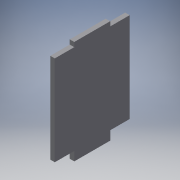
# Autodesk Inventor part: Base and top seperator
Saved by Autodesk Inventor 2018 (Build 220112000, 112)
## iProperties
Created: 2018-05-02
Part Number: Base and top seperator
Material: Generic
Document SubType Name: Modeling
Designer: Ajith Thomas
Density: 1 g/cm^3
Appearance: Default
Author: Ajith Thomas
Autodesk Inventor part; units mm, degrees
ref_plane "YZ Plane" through (0, 0, 0) normal (1, 0, 0) x (0, 1, 0)
ref_plane "XZ Plane" through (0, 0, 0) normal (0, 1, 0) x (-1, 0, 0)
ref_plane "XY Plane" through (0, 0, 0) normal (0, 0, 1) x (1, 0, 0)
sketch "Sketch1" plane through (0, 0, 0) normal (1, 0, 0) x (0, 1, 0)
  line L0 (30, 25) -> (-30, 25)
  line L1 (-30, 25) -> (-30, -25)
  line L2 (-30, -25) -> (30, -25)
  line L3 (30, -25) -> (30, 25)
  line L4 (30, 25) -> (-30, -25) construction
  line L5 (-30, 25) -> (30, -25) construction
  line L6 (36, 12) -> (30, 12)
  line L7 (30, 12) -> (30, -12)
  line L8 (30, -12) -> (36, -12)
  line L9 (36, -12) -> (36, 12)
  line L10 (0, 25) -> (0, -25) construction
  line L11 (-36, 12) -> (-30, 12)
  line L12 (-30, 12) -> (-30, -12)
  line L13 (-30, -12) -> (-36, -12)
  line L14 (-36, -12) -> (-36, 12)
  point P0 (0, 0)
  dimension "d0" = 60
  dimension "d1" = 50
  dimension "d2" = 6
  dimension "d3" = 13
  dimension "d4" = 13
  dimension "d5" = 24
  constraints: 30 end point, 4 midpoint, 4 parallel, 4 symmetric about line, 2 horizontal, 2 perpendicular, 1 point on line
  measures "d0" distance of L2.end L1.end
  measures "d1" distance of L1.end L0.end
  measures "d2" distance between parallel lines of L3 L9
  measures "d3" distance between parallel lines of L0 L6
  measures "d4" distance between parallel lines of L2 L8
  measures "d5" distance between parallel lines of L8 L6
extrude "Extrusion1" add sketch "Sketch1" along normal blind 3
sketch "Sketch2" plane through (3, 0, 0) normal (1, 0, 0) x (0, 0, -1)
  line L0 (12, 36) -> (-12, 36) projected
  line L1 (-12, 36) -> (-12, 30) projected
  line L2 (12, 30) -> (12, 36) projected
  line L3 (-12, 36) -> (-12, 30) projected
  line L4 (-12, 33) -> (12, 33)
  point P0 (0, 0)
  dimension "d8" = 3
  constraints: 2 end point, 2 midpoint
  measures "d8" distance between parallel lines of L0 L4
extrude "Extrusion2" cut sketch "Sketch2" against normal blind 3
body "Solid1"
